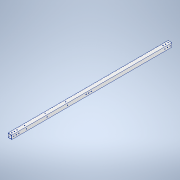
# Autodesk Inventor part: オムニ_角柱8
Saved by Autodesk Inventor 2021 (Build 250183000, 183)
## iProperties
Created: 2022-02-03
Part Number: オムニ_角柱8
Material: アルミニウム 6061
Document SubType Name: Modeling
Designer: hirohumi
Density: 2.7 g/cm^3
Appearance: アルミニウム - フラット
Mass: 93.8486 g
Surface Area: 699.31 cm^2
Volume: 34.7587 cm^3
Author: hirohumi
Autodesk Inventor part; units mm, degrees
ref_plane "YZ Plane" through (0, 0, 0) normal (1, 0, 0) x (0, 1, 0)
ref_plane "XZ Plane" through (0, 0, 0) normal (0, 1, 0) x (-1, 0, 0)
ref_plane "XY Plane" through (0, 0, 0) normal (0, 0, 1) x (1, 0, 0)
sketch "スケッチ1" plane through (0, 0, 0) normal (0, 0, 1) x (1, 0, 0)
  line L0 (7.5, 7.5) -> (-7.5, 7.5)
  line L1 (-7.5, 7.5) -> (-7.5, -7.5)
  line L2 (-7.5, -7.5) -> (7.5, -7.5)
  line L3 (7.5, -7.5) -> (7.5, 7.5)
  line L4 (7.5, 7.5) -> (-7.5, -7.5) construction
  line L5 (-7.5, 7.5) -> (7.5, -7.5) construction
  line L6 (-6.5, 6.5) -> (6.5, 6.5)
  line L7 (6.5, 6.5) -> (6.5, -6.5)
  line L8 (6.5, -6.5) -> (-6.5, -6.5)
  line L9 (-6.5, -6.5) -> (-6.5, 6.5)
  point P0 (0, 0)
  dimension "d0" = 15
  dimension "d1" = 15
  dimension "d2" = 1
  constraints: 20 end point, 4 parallel, 2 midpoint, 2 perpendicular, 1 horizontal, 3 other
  measures "d0" distance of L2.end L1.end
  measures "d1" distance of L1.end L0.end
  measures "d2" distance between parallel lines of L0 L6
extrude "押し出し1" add sketch "スケッチ1" along normal blind 625
sketch "スケッチ2" plane through (7.5, -7.5, 0) normal (1, 0, 0) x (0, 0, -1)
  circle A0 centre (-7.5, 7.5) radius 1.6
  circle A1 centre (-17.5, 7.5) radius 1.6
  circle A2 centre (-27.5, 7.5) radius 1.6
  line L0 (0, 0) -> (0, 15) projected
  circle A3 centre (-597.5, 7.5) radius 1.6
  circle A4 centre (-607.5, 7.5) radius 1.6
  circle A5 centre (-617.5, 7.5) radius 1.6
  line L1 (-625, 0) -> (-625, 15) projected
  circle A6 centre (-315, 7.5) radius 1.6
  circle A7 centre (-325, 7.5) radius 1.6
  circle A8 centre (-335, 7.5) radius 1.6
  circle A9 centre (-567.5, 7.5) radius 1.6
  circle A10 centre (-487.5, 7.5) radius 1.5
  circle A11 centre (-407.5, 7.5) radius 1.6
  point P0 (0, 7.5)
  point P1 (0, 7.5)
  point P2 (-625, 7.5)
  dimension "d5" = 3.2
  dimension "d6" = 3.2
  dimension "d7" = 3.2
  dimension "d8" = 7.5
  dimension "d9" = 10
  dimension "d10" = 10
  dimension "d13" = 3.2
  dimension "d14" = 3.2
  dimension "d15" = 3.2
  dimension "d16" = 10
  dimension "d17" = 10
  dimension "d18" = 7.5
  dimension "d40" = 3.2
  dimension "d41" = 3.2
  dimension "d42" = 3.2
  dimension "d43" = 10
  dimension "d44" = 10
  dimension "d45" = 300
  dimension "d52" = 3.2
  dimension "d53" = 3
  dimension "d54" = 3.2
  dimension "d55" = 80
  dimension "d56" = 80
  dimension "d57" = 30
  constraints: 12 centre point, 12 horizontal alignment, 2 midpoint
  measures "d5" diameter of A0
  measures "d6" diameter of A1
  measures "d7" diameter of A2
  measures "d8" distance of point (0, 7.5) A0.centre
  measures "d9" distance of A0.centre A1.centre
  measures "d10" distance of A1.centre A2.centre
  measures "d13" diameter of A3
  measures "d14" diameter of A4
  measures "d15" diameter of A5
  measures "d16" distance of A3.centre A4.centre
  measures "d17" distance of A4.centre A5.centre
  measures "d18" distance from line of A5.centre L1
  measures "d40" diameter of A6
  measures "d41" diameter of A7
  measures "d42" diameter of A8
  measures "d43" distance of A6.centre A7.centre
  measures "d44" distance of A7.centre A8.centre
  measures "d45" distance of A7.centre point (-625, 7.5)
  measures "d52" diameter of A9
  measures "d53" diameter of A10
  measures "d54" diameter of A11
  measures "d55" distance of A10.centre A9.centre
  measures "d56" distance of A11.centre A10.centre
  measures "d57" distance of A9.centre A3.centre
extrude "押し出し2" cut sketch "スケッチ2" against normal through all
sketch "スケッチ3" plane through (-7.5, 7.5, 0) normal (0, 1, 0) x (1, 0, 0)
  circle A0 centre (7.5, -17.5) radius 1.6
  circle A1 centre (7.5, -27.5) radius 1.6
  circle A2 centre (7.5, -597.5) radius 1.6
  circle A3 centre (7.5, -607.5) radius 1.6
  circle A4 centre (7.5, -617.5) radius 1.6
  line L0 (15, 0) -> (0, 0) projected
  circle A5 centre (7.5, -7.5) radius 1.6
  line L1 (15, -625) -> (0, -625) projected
  circle A6 centre (7.5, -407.5) radius 1.6
  circle A7 centre (7.5, -487.5) radius 1.5
  circle A8 centre (7.5, -567.5) radius 1.6
  point P0 (7.5, 0)
  dimension "d22" = 3.2
  dimension "d23" = 3.2
  dimension "d26" = 10
  dimension "d27" = 3.2
  dimension "d28" = 3.2
  dimension "d29" = 3.2
  dimension "d30" = 10
  dimension "d31" = 10
  dimension "d33" = 3.2
  dimension "d34" = 7.5
  dimension "d35" = 10
  dimension "d36" = 7.5
  dimension "d46" = 3.2
  dimension "d47" = 3
  dimension "d48" = 3.2
  dimension "d49" = 80
  dimension "d50" = 80
  dimension "d51" = 30
  constraints: 9 centre point, 9 vertical alignment, 1 midpoint
  measures "d22" diameter of A0
  measures "d23" diameter of A1
  measures "d26" distance of A0.centre A1.centre
  measures "d27" diameter of A2
  measures "d28" diameter of A3
  measures "d29" diameter of A4
  measures "d30" distance of A2.centre A3.centre
  measures "d31" distance of A3.centre A4.centre
  measures "d33" diameter of A5
  measures "d34" distance of A5.centre point (7.5, 0)
  measures "d35" distance of A5.centre A0.centre
  measures "d36" distance from line of A4.centre L1
  measures "d46" diameter of A6
  measures "d47" diameter of A7
  measures "d48" diameter of A8
  measures "d49" distance of A7.centre A6.centre
  measures "d50" distance of A8.centre A7.centre
  measures "d51" distance of A2.centre A8.centre
extrude "押し出し3" cut sketch "スケッチ3" against normal through all
